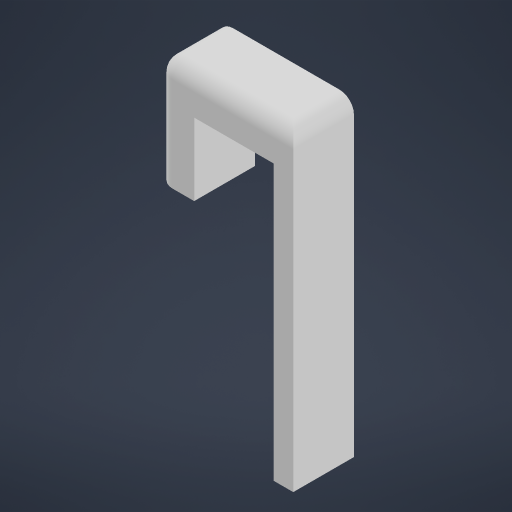
# Autodesk Inventor part: Hook_TestFit
Saved by Autodesk Inventor 2024.1 (Build 281209000, 209)
## iProperties
Created: 2023-07-11
Part Number: Hook_TestFit
Material: Generic
Document SubType Name: Modeling
Designer: User
Density: 1 g/cm^3
Appearance: Default
Author: User
Autodesk Inventor part; units mm, degrees
ref_plane "YZ Plane" through (0, 0, 0) normal (1, 0, 0) x (0, 1, 0)
ref_plane "XZ Plane" through (0, 0, 0) normal (0, 1, 0) x (-1, 0, 0)
ref_plane "XY Plane" through (0, 0, 0) normal (0, 0, 1) x (1, 0, 0)
sketch "Sketch1" plane through (0, 0, 0) normal (0, 0, 1) x (1, 0, 0)
  line L0 (0, 0) -> (-8.7, 0)
  line L1 (-8.7, 0) -> (-8.7, 8.7)
  line L2 (-8.7, 8.7) -> (0, 8.7)
  line L3 (0, 8.7) -> (0, 0)
  dimension "d0" = 8.7
  dimension "d1" = 8.7
  constraints: 8 end point, 2 parallel, 1 horizontal, 1 perpendicular
  measures "d0" distance of L1.end L2.end
  measures "d1" distance of L0.end L1.end
extrude "Extrusion1" [suppressed]
sketch "Sketch2" plane through (-8.7, 0, 0) normal (-1, 0, 0) x (0, 0, 1)
  line L0 (0, 8.7) -> (0, 0) projected
  line L1 (0, 0) -> (3, 0)
  line L2 (3, 0) -> (3, 8.7)
  line L3 (3, 8.7) -> (0, 8.7)
  line L4 (0, 8.7) -> (0, 0)
  constraints: 8 end point, 2 parallel, 1 horizontal, 1 perpendicular
extrude "Extrusion2" [suppressed]
sketch "Sketch3" plane through (0, 0, 3) normal (0, 0, 1) x (1, 0, 0)
  line L0 (0, 8.7) -> (-11.7, 8.7) projected
  line L1 (0, 0) -> (-11.7, 0) projected
  line L2 (-11.7, 8.7) -> (-8.7, 8.7)
  line L3 (-8.7, 8.7) -> (-8.7, 0)
  line L4 (-8.7, 0) -> (-11.7, 0)
  line L5 (-11.7, 0) -> (-11.7, 8.7)
  dimension "d6" = 3
  constraints: 8 end point, 2 parallel, 1 horizontal, 1 perpendicular, 1 point on line
  measures "d6" distance of L3.end L4.end
extrude "Extrusion3" [suppressed]
sketch "Sketch5" plane through (0, 0, 0) normal (1, 0, 0) x (0, 0, -1)
  line L0 (0, 8.7) -> (-3, 8.7) projected
  line L1 (0, 0) -> (-3, 0)
  line L2 (-3, 0) -> (-3, 8.7)
  line L3 (-3, 8.7) -> (0, 8.7)
  line L4 (0, 8.7) -> (0, 0)
  dimension "d9" = 3
  constraints: 8 end point, 2 parallel, 1 horizontal, 1 perpendicular
  measures "d9" distance of L0.end L3.end
extrude "Extrusion4" [suppressed]
sketch "Sketch6" plane through (0, 0, 3) normal (0, 0, 1) x (1, 0, 0)
  line L0 (3, 8.7) -> (-11.7, 8.7) projected
  line L1 (3, 8.7) -> (0, 8.7)
  line L2 (0, 8.7) -> (0, 0)
  line L3 (0, 0) -> (3, 0)
  line L4 (3, 0) -> (3, 8.7)
  constraints: 8 end point, 2 parallel, 1 horizontal, 1 perpendicular
extrude "Extrusion5" [suppressed]
sketch "Sketch7" plane through (0, 0, 0) normal (0, 0, 1) x (1, 0, 0)
  line L0 (0, 0) -> (-2.7, 0)
  line L1 (-2.7, 0) -> (-2.7, 43)
  line L2 (-2.7, 43) -> (0, 43)
  line L3 (0, 43) -> (0, 0)
  line L4 (-2.7, 43) -> (-13.7, 43)
  line L5 (-13.7, 43) -> (-13.7, 38)
  line L6 (-13.7, 38) -> (-2.7, 38)
  line L7 (-2.7, 38) -> (-2.7, 43)
  line L8 (-13.7, 43) -> (-18.7, 43)
  line L9 (-18.7, 43) -> (-18.7, 28)
  line L10 (-18.7, 28) -> (-13.7, 28)
  line L11 (-13.7, 28) -> (-13.7, 43)
  point P0 (-2.7, 38)
  dimension "d14" = 2.7
  dimension "d15" = 43
  dimension "d16" = 11
  dimension "d17" = 5
  dimension "d18" = 5
  dimension "d19" = 15
  constraints: 24 end point, 6 parallel, 3 horizontal, 3 perpendicular
  measures "d14" distance of L1.end L2.end
  measures "d15" distance of L0.end L1.end
  measures "d16" distance of L6.end L5.end
  measures "d17" distance of L5.end L4.end
  measures "d18" distance of L10.end L9.end
  measures "d19" distance of L9.end L8.end
extrude "Extrusion6" add sketch "Sketch7" along normal blind 8.4
fillet "Fillet1" radius 2 6 edges at (-18.7, 35.5, 8.4) (-16.2, 43, 8.4) (-8.2, 43, 8.4) (-1.35, 43, 8.4) (0, 43, 4.2) (-18.7, 43, 4.2)
body "Solid1"
